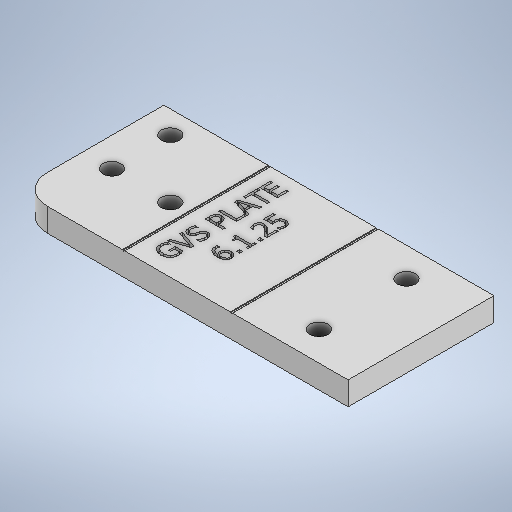
# Autodesk Inventor part: GVS_.Mount
Saved by Autodesk Inventor 2025 (Build 290162000, 162)
## iProperties
Created: 2025-05-19
Part Number: GVS_.Mount
Material: Generic
Document SubType Name: Modeling
Designer: mumin
Density: 1 g/cm^3
Appearance: Default
Author: mumin
Autodesk Inventor part; units mm, degrees
ref_plane "YZ Plane" through (0, 0, 0) normal (1, 0, 0) x (0, 1, 0)
ref_plane "XZ Plane" through (0, 0, 0) normal (0, 1, 0) x (-1, 0, 0)
ref_plane "XY Plane" through (0, 0, 0) normal (0, 0, 1) x (1, 0, 0)
sketch "Sketch1" plane through (0, 0, 0) normal (0, 1, 0) x (-1, 0, 0)
  line L0 (10.5834, 13.2197) -> (-45.9966, 13.2197)
  line L1 (-45.9966, 13.2197) -> (-45.9966, -11.7803)
  line L2 (-45.9966, -11.7803) -> (10.5834, -11.7803)
  line L3 (10.5834, -11.7803) -> (10.5834, 13.2197)
  circle A0 centre (5.5834, -7.8803) radius 1.55
  circle A1 centre (5.5834, 2.1197) radius 1.55
  circle A2 centre (-4.4166, 2.1197) radius 1.55
  circle A3 centre (-35.9966, 8.2197) radius 1.55
  circle A4 centre (-35.9966, -6.7803) radius 1.55
  point P0 (0, 0)
  dimension "d0" = 3.1
  dimension "d1" = 3.9
  dimension "d4" = 10
  dimension "d11" = 10
  dimension "d16" = 25
  dimension "d17" = 5
  dimension "d18" = 56.58
  dimension "d19" = 3.1
  dimension "d20" = 10
  dimension "d23" = 15
  dimension "d28" = 5
  constraints: 8 end point, 5 centre point, 2 horizontal, 2 parallel, 2 vertical, 1 perpendicular, 6 other
  measures "d0" diameter of A0
  measures "d1" distance from line of L2 A0.centre
  measures "d4" distance of A0.centre A1.centre
  measures "d11" distance of A1.centre A2.centre
  measures "d16" distance of L2.end L0.start
  measures "d17" distance from line of L3 A0.centre
  measures "d18" distance of L0.start L0.end
  measures "d19" diameter of A3
  measures "d20" distance from line of L1 A3.centre
  measures "d23" distance of A3.centre A4.centre
  measures "d28" distance from line of A3.centre L0
extrude "Extrusion1" add sketch "Sketch1" along normal mid plane 4
sketch "Sketch2" plane through (45.9966, 2, -11.7803) normal (0, 0, -1) x (-1, 0, 0)
  arc A0 (38.37, 0) -> (38.62, 0) centre (38.495, 0) ccw
  line L0 (0, 0) -> (56.58, 0) projected
  line L1 (56.58, -4) -> (56.58, 0) projected
  circle A1 centre (20, 0) radius 0.125
  line L2 (0, -4) -> (0, 0) projected
  point P0 (45.9966, -2)
  point P1 (56.58, -2)
  point P2 (20.125, 0)
  point P3 (19.875, 0)
  dimension "d31" = 0.25
  dimension "d34" = 18.085
  dimension "d35" = 0.25
  dimension "d36" = 20
  constraints: 4 point on line, 2 centre point, 2 point on circle, 1 midpoint
  measures "d31" diameter of A0
  measures "d34" horizontal distance of point (56.58, -2) A0.centre
  measures "d35" diameter of A1
  measures "d36" distance from line of L2 A1.centre
extrude "Extrusion2" cut sketch "Sketch2" against normal up to surface (25 mm away) contours L0 A0 | L0 A1 picked at (20, -0.0736)
fillet "Fillet1" radius 0.1 4 edges at (7.3766, 2, 0.7197) (7.6266, 2, 0.7197) (25.8716, 2, 0.7197) (26.1216, 2, 0.7197)
fillet "Fillet2" radius 5 1 edges at (-10.5834, 0, 13.2197)
sketch "Sketch3" plane through (0, 2, 0) normal (0, 1, 0) x (1, 0, 0)
  line L0 (9.7955, -15.9747) -> (9.7955, 14.94) construction
  line L1 (9.7955, 14.94) -> (23.0854, 14.94) construction
  line L2 (23.0854, 14.94) -> (23.0854, -15.9747) construction
  line L3 (23.0854, -15.9747) -> (9.7955, -15.9747) construction
  spline S0 degree 2 poles (12.9571, -9.2587) (12.9571, -9.5823) (12.7595, -10.1183) (12.5594, -10.311) knots 0 0 0 1 2 2 2
  spline S1 degree 2 poles (12.5594, -10.311) (12.3569, -10.5036) (11.7591, -10.7086) (11.3713, -10.7086) knots 0 0 0 1 2 2 2
  spline S2 degree 2 poles (11.3713, -10.7086) (11.0033, -10.7086) (10.4204, -10.5011) (10.2129, -10.3085) knots 0 0 0 1 2 2 2
  spline S3 degree 2 poles (10.2129, -10.3085) (10.0128, -10.1232) (9.7955, -9.5798) (9.7955, -9.2563) knots 0 0 0 1 2 2 2
  spline S4 degree 2 poles (9.7955, -9.2563) (9.7955, -9.1006) (9.8399, -8.8191) (9.8795, -8.6906) knots 0 0 0 1 2 2 2
  spline S5 degree 2 poles (9.8795, -8.6906) (9.9091, -8.5869) (10.0178, -8.3349) (10.0573, -8.2584) knots 0 0 0 1 2 2 2
  line L4 (10.0573, -8.2584) -> (10.5464, -8.2584)
  line L5 (10.5464, -8.2584) -> (10.5464, -8.293)
  spline S6 degree 2 poles (10.5464, -8.293) (10.4797, -8.3695) (10.3586, -8.5301) (10.2895, -8.6783) knots 0 0 0 1 2 2 2
  spline S7 degree 2 poles (10.2895, -8.6783) (10.2277, -8.8018) (10.1462, -9.1204) (10.1462, -9.3032) knots 0 0 0 1 2 2 2
  spline S8 degree 2 poles (10.1462, -9.3032) (10.1462, -9.7429) (10.8082, -10.2863) (11.359, -10.2863) knots 0 0 0 1 2 2 2
  spline S9 degree 2 poles (11.359, -10.2863) (11.6653, -10.2863) (12.1247, -10.143) (12.2828, -10.0071) knots 0 0 0 1 2 2 2
  spline S10 degree 2 poles (12.2828, -10.0071) (12.4409, -9.8762) (12.6064, -9.5057) (12.6064, -9.2735) knots 0 0 0 1 2 2 2
  spline S11 degree 2 poles (12.6064, -9.2735) (12.6064, -9.1031) (12.557, -8.7623) (12.5076, -8.6462) knots 0 0 0 1 2 2 2
  line L6 (12.5076, -8.6462) -> (11.7196, -8.6462)
  line L7 (11.7196, -8.6462) -> (11.7196, -9.3526)
  line L8 (11.7196, -9.3526) -> (11.3639, -9.3526)
  line L9 (11.3639, -9.3526) -> (11.3639, -8.246)
  line L10 (11.3639, -8.246) -> (12.6953, -8.246)
  spline S12 degree 2 poles (12.6953, -8.246) (12.7299, -8.3226) (12.8361, -8.5844) (12.8682, -8.6956) knots 0 0 0 1 2 2 2
  spline S13 degree 2 poles (12.8682, -8.6956) (12.9126, -8.8462) (12.9571, -9.0883) (12.9571, -9.2587) knots 0 0 0 1 2 2 2
  line L11 (9.8498, -5.5265) -> (12.8978, -6.5763)
  line L12 (12.8978, -6.5763) -> (12.8978, -7.0135)
  line L13 (12.8978, -7.0135) -> (9.8498, -8.0632)
  line L14 (9.8498, -8.0632) -> (9.8498, -7.6285)
  line L15 (9.8498, -7.6285) -> (12.3816, -6.7838)
  line L16 (12.3816, -6.7838) -> (9.8498, -5.939)
  line L17 (9.8498, -5.939) -> (9.8498, -5.5265)
  spline S14 degree 2 poles (12.9522, -4.3854) (12.9522, -4.7164) (12.8138, -5.1807) (12.715, -5.3857) knots 0 0 0 1 2 2 2
  line L18 (12.715, -5.3857) -> (12.2062, -5.3857)
  line L19 (12.2062, -5.3857) -> (12.2062, -5.3561)
  spline S15 degree 2 poles (12.2062, -5.3561) (12.3939, -5.156) (12.6014, -4.6497) (12.6014, -4.415) knots 0 0 0 1 2 2 2
  spline S16 degree 2 poles (12.6014, -4.415) (12.6014, -4.0791) (12.3223, -3.7358) (12.0926, -3.7358) knots 0 0 0 1 2 2 2
  spline S17 degree 2 poles (12.0926, -3.7358) (11.9098, -3.7358) (11.6826, -3.9161) (11.6258, -4.1112) knots 0 0 0 1 2 2 2
  spline S18 degree 2 poles (11.6258, -4.1112) (11.5862, -4.252) (11.5319, -4.4867) (11.4874, -4.662) knots 0 0 0 1 2 2 2
  spline S19 degree 2 poles (11.4874, -4.662) (11.4454, -4.8201) (11.3195, -5.0696) (11.2182, -5.1659) knots 0 0 0 1 2 2 2
  spline S20 degree 2 poles (11.2182, -5.1659) (11.1169, -5.2598) (10.8452, -5.3635) (10.6674, -5.3635) knots 0 0 0 1 2 2 2
  spline S21 degree 2 poles (10.6674, -5.3635) (10.2969, -5.3635) (9.7955, -4.7855) (9.7955, -4.3385) knots 0 0 0 1 2 2 2
  spline S22 degree 2 poles (9.7955, -4.3385) (9.7955, -4.0816) (9.8967, -3.6271) (9.9931, -3.432) knots 0 0 0 1 2 2 2
  line L20 (9.9931, -3.432) -> (10.4772, -3.432)
  line L21 (10.4772, -3.432) -> (10.4772, -3.4616)
  spline S23 degree 2 poles (10.4772, -3.4616) (10.3438, -3.6073) (10.1462, -4.0618) (10.1462, -4.3113) knots 0 0 0 1 2 2 2
  spline S24 degree 2 poles (10.1462, -4.3113) (10.1462, -4.5929) (10.4105, -4.9411) (10.6254, -4.9411) knots 0 0 0 1 2 2 2
  spline S25 degree 2 poles (10.6254, -4.9411) (10.8181, -4.9411) (11.0478, -4.7361) (11.0996, -4.5435) knots 0 0 0 1 2 2 2
  spline S26 degree 2 poles (11.0996, -4.5435) (11.1342, -4.415) (11.2231, -4.0421) (11.2602, -3.9186) knots 0 0 0 1 2 2 2
  spline S27 degree 2 poles (11.2602, -3.9186) (11.3565, -3.6049) (11.7443, -3.3134) (12.0284, -3.3134) knots 0 0 0 1 2 2 2
  spline S28 degree 2 poles (12.0284, -3.3134) (12.2087, -3.3134) (12.5545, -3.4591) (12.6755, -3.59) knots 0 0 0 1 2 2 2
  spline S29 degree 2 poles (12.6755, -3.59) (12.8089, -3.7358) (12.9522, -4.1063) (12.9522, -4.3854) knots 0 0 0 1 2 2 2
  spline S30 degree 2 poles (10.7687, 0.3348) (10.9663, 0.3348) (11.3219, 0.194) (11.4454, 0.0681) knots 0 0 0 1 2 2 2
  spline S31 degree 2 poles (11.4454, 0.0681) (11.6011, -0.09) (11.7616, -0.5173) (11.7616, -0.8434) knots 0 0 0 1 2 2 2
  line L22 (11.7616, -0.8434) -> (11.7616, -1.1867)
  line L23 (11.7616, -1.1867) -> (12.8978, -1.1867)
  line L24 (12.8978, -1.1867) -> (12.8978, -1.5918)
  line L25 (12.8978, -1.5918) -> (9.8498, -1.5918)
  line L26 (9.8498, -1.5918) -> (9.8498, -0.8261)
  spline S32 degree 2 poles (9.8498, -0.8261) (9.8498, -0.5544) (9.9387, -0.174) (10.04, -0.0283) knots 0 0 0 1 2 2 2
  spline S33 degree 2 poles (10.04, -0.0283) (10.1561, 0.1422) (10.5143, 0.3348) (10.7687, 0.3348) knots 0 0 0 1 2 2 2
  spline S34 degree 2 poles (10.781, -0.0876) (10.6229, -0.0876) (10.3908, -0.1962) (10.3166, -0.3074) knots 0 0 0 1 2 2 2
  spline S35 degree 2 poles (10.3166, -0.3074) (10.2524, -0.4037) (10.2006, -0.6606) (10.2006, -0.8508) knots 0 0 0 1 2 2 2
  line L27 (10.2006, -0.8508) -> (10.2006, -1.1867)
  line L28 (10.2006, -1.1867) -> (11.4158, -1.1867)
  line L29 (11.4158, -1.1867) -> (11.4158, -0.9101)
  spline S36 degree 2 poles (11.4158, -0.9101) (11.4158, -0.6631) (11.3368, -0.3593) (11.233, -0.2605) knots 0 0 0 1 2 2 2
  spline S37 degree 2 poles (11.233, -0.2605) (11.1416, -0.1691) (10.9267, -0.0876) (10.781, -0.0876) knots 0 0 0 1 2 2 2
  line L30 (12.8978, 2.4862) -> (12.8978, 0.7201)
  line L31 (12.8978, 0.7201) -> (9.8498, 0.7201)
  line L32 (9.8498, 0.7201) -> (9.8498, 1.1252)
  line L33 (9.8498, 1.1252) -> (12.5372, 1.1252)
  line L34 (12.5372, 1.1252) -> (12.5372, 2.4862)
  line L35 (12.5372, 2.4862) -> (12.8978, 2.4862)
  line L36 (12.8978, 2.4763) -> (9.8498, 3.5038)
  line L37 (9.8498, 3.5038) -> (9.8498, 4.0028)
  line L38 (9.8498, 4.0028) -> (12.8978, 5.0303)
  line L39 (12.8978, 5.0303) -> (12.8978, 4.603)
  line L40 (12.8978, 4.603) -> (12.0457, 4.3264)
  line L41 (12.0457, 4.3264) -> (12.0457, 3.163)
  line L42 (12.0457, 3.163) -> (12.8978, 2.8863)
  line L43 (12.8978, 2.8863) -> (12.8978, 2.4763)
  line L44 (11.6999, 4.2152) -> (10.2648, 3.7434)
  line L45 (10.2648, 3.7434) -> (11.6999, 3.2741)
  line L46 (11.6999, 3.2741) -> (11.6999, 4.2152)
  line L47 (12.8978, 6.0307) -> (10.2104, 6.0307)
  line L48 (10.2104, 6.0307) -> (10.2104, 5.0081)
  line L49 (10.2104, 5.0081) -> (9.8498, 5.0081)
  line L50 (9.8498, 5.0081) -> (9.8498, 7.4583)
  line L51 (9.8498, 7.4583) -> (10.2104, 7.4583)
  line L52 (10.2104, 7.4583) -> (10.2104, 6.4358)
  line L53 (10.2104, 6.4358) -> (12.8978, 6.4358)
  line L54 (12.8978, 6.4358) -> (12.8978, 6.0307)
  line L55 (12.8978, 7.7671) -> (9.8498, 7.7671)
  line L56 (9.8498, 7.7671) -> (9.8498, 9.6739)
  line L57 (9.8498, 9.6739) -> (10.2104, 9.6739)
  line L58 (10.2104, 9.6739) -> (10.2104, 8.1722)
  line L59 (10.2104, 8.1722) -> (11.0453, 8.1722)
  line L60 (11.0453, 8.1722) -> (11.0453, 9.5727)
  line L61 (11.0453, 9.5727) -> (11.4059, 9.5727)
  line L62 (11.4059, 9.5727) -> (11.4059, 8.1722)
  line L63 (11.4059, 8.1722) -> (12.5372, 8.1722)
  line L64 (12.5372, 8.1722) -> (12.5372, 9.6739)
  line L65 (12.5372, 9.6739) -> (12.8978, 9.6739)
  line L66 (12.8978, 9.6739) -> (12.8978, 7.7671)
  spline S38 degree 2 poles (16.9283, -4.2125) (17.1629, -4.2125) (17.5606, -4.3681) (17.694, -4.499) knots 0 0 0 1 2 2 2
  spline S39 degree 2 poles (17.694, -4.499) (17.8348, -4.6349) (17.9805, -4.9757) (17.9805, -5.1807) knots 0 0 0 1 2 2 2
  spline S40 degree 2 poles (17.9805, -5.1807) (17.9805, -5.3857) (17.8422, -5.7241) (17.7038, -5.8526) knots 0 0 0 1 2 2 2
  spline S41 degree 2 poles (17.7038, -5.8526) (17.5384, -6.0107) (16.9826, -6.1885) (16.5775, -6.1885) knots 0 0 0 1 2 2 2
  spline S42 degree 2 poles (16.5775, -6.1885) (16.1798, -6.1885) (15.5401, -6.0255) (15.303, -5.855) knots 0 0 0 1 2 2 2
  spline S43 degree 2 poles (15.303, -5.855) (15.0708, -5.6896) (14.8115, -5.1659) (14.8115, -4.8226) knots 0 0 0 1 2 2 2
  spline S44 degree 2 poles (14.8115, -4.8226) (14.8115, -4.7213) (14.8312, -4.5435) (14.8534, -4.4768) knots 0 0 0 1 2 2 2
  line L67 (14.8534, -4.4768) -> (15.2462, -4.4768)
  line L68 (15.2462, -4.4768) -> (15.2462, -4.4941)
  spline S45 degree 2 poles (15.2462, -4.4941) (15.2165, -4.5509) (15.1647, -4.7584) (15.1647, -4.8769) knots 0 0 0 1 2 2 2
  spline S46 degree 2 poles (15.1647, -4.8769) (15.1647, -5.2573) (15.6784, -5.7241) (16.1823, -5.7686) knots 0 0 0 1 2 2 2
  spline S47 degree 2 poles (16.1823, -5.7686) (16.081, -5.6229) (15.9699, -5.3166) (15.9699, -5.1338) knots 0 0 0 1 2 2 2
  spline S48 degree 2 poles (15.9699, -5.1338) (15.9699, -4.956) (16.0415, -4.6892) (16.1502, -4.5435) knots 0 0 0 1 2 2 2
  spline S49 degree 2 poles (16.1502, -4.5435) (16.2762, -4.3755) (16.6664, -4.2125) (16.9283, -4.2125) knots 0 0 0 1 2 2 2
  spline S50 degree 2 poles (16.9456, -4.6274) (16.7578, -4.6274) (16.5034, -4.7262) (16.4145, -4.8349) knots 0 0 0 1 2 2 2
  spline S51 degree 2 poles (16.4145, -4.8349) (16.3503, -4.9164) (16.3083, -5.119) (16.3083, -5.2252) knots 0 0 0 1 2 2 2
  spline S52 degree 2 poles (16.3083, -5.2252) (16.3083, -5.3685) (16.3947, -5.6377) (16.4762, -5.7686) knots 0 0 0 1 2 2 2
  spline S53 degree 2 poles (16.4762, -5.7686) (16.5207, -5.7711) (16.6047, -5.776) (16.6689, -5.776) knots 0 0 0 1 2 2 2
  spline S54 degree 2 poles (16.6689, -5.776) (16.9851, -5.776) (17.3729, -5.6525) (17.4741, -5.5586) knots 0 0 0 1 2 2 2
  spline S55 degree 2 poles (17.4741, -5.5586) (17.5705, -5.4722) (17.647, -5.2845) (17.647, -5.1783) knots 0 0 0 1 2 2 2
  spline S56 degree 2 poles (17.647, -5.1783) (17.647, -4.9313) (17.2963, -4.6274) (16.9456, -4.6274) knots 0 0 0 1 2 2 2
  line L69 (17.9163, -3.1973) -> (17.9163, -3.6864)
  line L70 (17.9163, -3.6864) -> (17.3333, -3.6864)
  line L71 (17.3333, -3.6864) -> (17.3333, -3.1973)
  line L72 (17.3333, -3.1973) -> (17.9163, -3.1973)
  line L73 (17.9163, -0.8557) -> (17.9163, -2.3427)
  line L74 (17.9163, -2.3427) -> (17.605, -2.3427)
  line L75 (17.605, -2.3427) -> (17.605, -1.7894)
  line L76 (17.605, -1.7894) -> (15.5623, -1.7894)
  line L77 (15.5623, -1.7894) -> (15.5623, -2.3427)
  line L78 (15.5623, -2.3427) -> (15.2832, -2.3427)
  spline S57 degree 2 poles (15.2832, -2.3427) (15.2832, -2.029) (15.1054, -1.7326) (14.8584, -1.7128) knots 0 0 0 1 2 2 2
  line L79 (14.8584, -1.7128) -> (14.8584, -1.3967)
  line L80 (14.8584, -1.3967) -> (17.605, -1.3967)
  line L81 (17.605, -1.3967) -> (17.605, -0.8557)
  line L82 (17.605, -0.8557) -> (17.9163, -0.8557)
  line L83 (17.9163, 0.3595) -> (17.9163, -0.1295)
  line L84 (17.9163, -0.1295) -> (17.3333, -0.1295)
  line L85 (17.3333, -0.1295) -> (17.3333, 0.3595)
  line L86 (17.3333, 0.3595) -> (17.9163, 0.3595)
  line L87 (17.9163, 2.8542) -> (17.9163, 0.9745)
  line L88 (17.9163, 0.9745) -> (17.484, 0.9745)
  spline S58 degree 2 poles (17.484, 0.9745) (17.2938, 1.1771) (16.9406, 1.5377) (16.7504, 1.7106) knots 0 0 0 1 2 2 2
  spline S59 degree 2 poles (16.7504, 1.7106) (16.3676, 2.0589) (15.9081, 2.3133) (15.6636, 2.3133) knots 0 0 0 1 2 2 2
  spline S60 degree 2 poles (15.6636, 2.3133) (15.5352, 2.3133) (15.3425, 2.2343) (15.2808, 2.1626) knots 0 0 0 1 2 2 2
  spline S61 degree 2 poles (15.2808, 2.1626) (15.219, 2.091) (15.1573, 1.9033) (15.1573, 1.7897) knots 0 0 0 1 2 2 2
  spline S62 degree 2 poles (15.1573, 1.7897) (15.1573, 1.681) (15.2116, 1.4587) (15.2536, 1.3574) knots 0 0 0 1 2 2 2
  spline S63 degree 2 poles (15.2536, 1.3574) (15.2882, 1.271) (15.387, 1.1104) (15.4216, 1.061) knots 0 0 0 1 2 2 2
  line L89 (15.4216, 1.061) -> (15.4216, 1.0388)
  line L90 (15.4216, 1.0388) -> (14.9868, 1.0388)
  spline S64 degree 2 poles (14.9868, 1.0388) (14.9251, 1.1647) (14.804, 1.6168) (14.804, 1.8193) knots 0 0 0 1 2 2 2
  spline S65 degree 2 poles (14.804, 1.8193) (14.804, 2.2466) (15.2561, 2.7283) (15.6414, 2.7283) knots 0 0 0 1 2 2 2
  spline S66 degree 2 poles (15.6414, 2.7283) (15.8217, 2.7283) (16.123, 2.6443) (16.2515, 2.5702) knots 0 0 0 1 2 2 2
  spline S67 degree 2 poles (16.2515, 2.5702) (16.3849, 2.4961) (16.6467, 2.2812) (16.7727, 2.1626) knots 0 0 0 1 2 2 2
  spline S68 degree 2 poles (16.7727, 2.1626) (16.9826, 1.97) (17.4321, 1.4982) (17.5631, 1.3574) knots 0 0 0 1 2 2 2
  line L91 (17.5631, 1.3574) -> (17.5631, 2.8542)
  line L92 (17.5631, 2.8542) -> (17.9163, 2.8542)
  spline S69 degree 2 poles (16.948, 5.1094) (17.1679, 5.1094) (17.5433, 4.9686) (17.6816, 4.8401) knots 0 0 0 1 2 2 2
  spline S70 degree 2 poles (17.6816, 4.8401) (17.8199, 4.7117) (17.9805, 4.3288) (17.9805, 4.0917) knots 0 0 0 1 2 2 2
  spline S71 degree 2 poles (17.9805, 4.0917) (17.9805, 3.8743) (17.8842, 3.4495) (17.8076, 3.2939) knots 0 0 0 1 2 2 2
  line L93 (17.8076, 3.2939) -> (17.3753, 3.2939)
  line L94 (17.3753, 3.2939) -> (17.3753, 3.3235)
  spline S72 degree 2 poles (17.3753, 3.3235) (17.4099, 3.3705) (17.4988, 3.5458) (17.5384, 3.652) knots 0 0 0 1 2 2 2
  spline S73 degree 2 poles (17.5384, 3.652) (17.5803, 3.7731) (17.6273, 3.9731) (17.6273, 4.0991) knots 0 0 0 1 2 2 2
  spline S74 degree 2 poles (17.6273, 4.0991) (17.6273, 4.2226) (17.5384, 4.4548) (17.442, 4.5388) knots 0 0 0 1 2 2 2
  spline S75 degree 2 poles (17.442, 4.5388) (17.3506, 4.6154) (17.1086, 4.6944) (16.9456, 4.6944) knots 0 0 0 1 2 2 2
  spline S76 degree 2 poles (16.9456, 4.6944) (16.7825, 4.6944) (16.575, 4.6055) (16.5059, 4.5215) knots 0 0 0 1 2 2 2
  spline S77 degree 2 poles (16.5059, 4.5215) (16.4293, 4.435) (16.3651, 4.1782) (16.3651, 4.0225) knots 0 0 0 1 2 2 2
  spline S78 degree 2 poles (16.3651, 4.0225) (16.3651, 3.8546) (16.417, 3.5211) (16.4392, 3.4199) knots 0 0 0 1 2 2 2
  line L95 (16.4392, 3.4199) -> (14.8683, 3.4199)
  line L96 (14.8683, 3.4199) -> (14.8683, 5.0921)
  line L97 (14.8683, 5.0921) -> (15.2264, 5.0921)
  line L98 (15.2264, 5.0921) -> (15.2264, 3.8126)
  line L99 (15.2264, 3.8126) -> (16.0391, 3.8126)
  spline S79 degree 2 poles (16.0391, 3.8126) (16.0292, 3.8867) (16.0218, 4.03) (16.0218, 4.0892) knots 0 0 0 1 2 2 2
  spline S80 degree 2 poles (16.0218, 4.0892) (16.0218, 4.3239) (16.0983, 4.6475) (16.212, 4.7957) knots 0 0 0 1 2 2 2
  spline S81 degree 2 poles (16.212, 4.7957) (16.3256, 4.9463) (16.6714, 5.1094) (16.948, 5.1094) knots 0 0 0 1 2 2 2
  point P0 (0, 0)
  constraints: 2 other
emboss "Emboss1" sketch "Sketch3" operation cut depth 1 direction (0, -1, 0)
body "Solid1"
